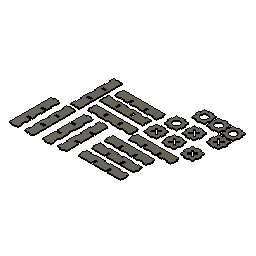
Verkefni2 (Autodesk Fusion 360 design; units mm, degrees)
Autodesk Fusion 360 part; units mm, degrees
note: some values were not read from the file. Chosen so that the rebuilt part matches the saved one: which bodies a step acts on. Set by a fixed rule: which sketch regions a step uses.
(part 1 of 6)
sketch "Rammi_lengd1_sketch" plane through (0, 0, 0) normal (1, 0, 0) x (0, 1, 0)
  line L0 (0, 0) -> (200, 0)
  line L1 (200, 0) -> (200, 40)
  line L2 (200, 40) -> (0, 40)
  line L3 (0, 40) -> (0, 0)
  dimension "d3" = 40
  dimension "d4" = 200
  constraint horizontal L0
  constraint vertical L1
  constraint horizontal L2
  constraint vertical L3
  constraint coincident L0.start L3.end
  measures "d3" distance of L0.start L2.end
  measures "d4" distance of L0.start L0.end
extrude "Extrude1" add sketch "Rammi_lengd1_sketch" along normal blind 4 makes body 1
sketch "V_Fingur_haed_sketch" plane through (0, 0, 0) normal (0, -1, 0) x (1, 0, 0)
  line L0 (0, 40) -> (0, 0)
  line L1 (0, 0) -> (4, 0)
  line L2 (4, 0) -> (4, 40)
  line L3 (4, 40) -> (0, 40)
  line L4 (0, 8) -> (4, 8)
  line L5 (4, 8) -> (4, 16)
  line L6 (4, 16) -> (0, 16)
  line L7 (0, 16) -> (0, 8)
  dimension "d13" = 8
  dimension "d14" = 8
  constraint horizontal L4
  constraint vertical L5
  constraint horizontal L6
  constraint vertical L7
  constraint coincident L2 L5.end
  constraint coincident L0 L4.start
  measures "d13" distance of L4.end L5.end
  measures "d14" distance of L1.end L4.end
extrude "Extrude2" cut sketch "V_Fingur_haed_sketch" against normal blind 4 contours L0 L2 L4 L5 L6 L7 bodies 1
pattern_linear "R-Pattern1" count 2 spacing 16 along (0, 0, 1) of "Extrude2"
sketch "Rammi_breidd_sketch" plane through (0, 0, 0) normal (0, 1, 0) x (1, 0, 0)
  line L0 (0, 0) -> (200, 0)
  line L1 (200, 0) -> (200, -40)
  line L2 (200, -40) -> (0, -40)
  line L3 (0, -40) -> (0, 0)
  dimension "d21" = 200
  dimension "d22" = 40
  constraint horizontal L0
  constraint vertical L1
  constraint horizontal L2
  constraint vertical L3
  constraint coincident L0.start L3.end
  measures "d21" distance of L1.end L2.end
  measures "d22" distance of L0.end L1.end
extrude "Extrude3" add sketch "Rammi_breidd_sketch" along normal blind 4 separate body makes body 2
combine "Combine1" operation cut target body 2 tool bodies 1 keep tools
extrude "Extrude4" add 1 faces at (4, 134.6667, 18.6667) along direction (-1, 0, 0) blind 4 from surface at -196 separate body on bodies 1 makes body 3
combine "Combine2" operation cut target body 2 tool bodies 3 keep tools
extrude "Extrude6" add 1 faces at (68, 4, 34.6667) along direction (0, -1, 0) blind 4 from surface at -196 separate body on bodies 2 makes body 4
combine "Combine4" operation cut target body 1 tool bodies 4 keep tools
combine "Combine7" operation cut target body 3 tool bodies 4 keep tools
sketch "got_a_hlidum1" plane through (0, 0, 0) normal (-1, 0, 0) x (0, -1, 0)
  line L0 (-196, 8) -> (-200, 8)
  line L1 (-200, 8) -> (-200, 0)
  line L2 (-200, 0) -> (0, 0)
  line L3 (0, 0) -> (0, 8)
  line L4 (0, 8) -> (-4, 8)
  line L5 (-4, 8) -> (-4, 16)
  line L6 (-4, 16) -> (0, 16)
  line L7 (0, 16) -> (0, 24)
  line L8 (0, 24) -> (-4, 24)
  line L9 (-4, 24) -> (-4, 32)
  line L10 (-4, 32) -> (0, 32)
  line L11 (0, 32) -> (0, 40)
  line L12 (0, 40) -> (-200, 40)
  line L13 (-200, 40) -> (-200, 32)
  line L14 (-200, 32) -> (-196, 32)
  line L15 (-196, 32) -> (-196, 24)
  line L16 (-196, 24) -> (-200, 24)
  line L17 (-200, 24) -> (-200, 16)
  line L18 (-200, 16) -> (-196, 16)
  line L19 (-196, 16) -> (-196, 8)
  line L20 (-137.3333, 28) -> (-129.3333, 28)
  line L21 (-129.3333, 28) -> (-129.3333, 12)
  line L22 (-129.3333, 12) -> (-137.3333, 12)
  line L23 (-137.3333, 12) -> (-137.3333, 28)
  dimension "d53" = 8
  dimension "d54" = 16
  dimension "d55" = 12
  dimension "d57" = 62.6667
  constraint horizontal L20
  constraint vertical L21
  constraint horizontal L22
  constraint vertical L23
  measures "d53" distance of L20.start L20.end
  measures "d54" distance of L20.end L21.end
  measures "d55" distance of L2 L22
  measures "d57" distance of L17 L23
extrude "Extrude8" cut sketch "got_a_hlidum1" against normal blind 4 contours L20 L21 L22 L23 bodies 1
sketch "got_a_hlidum2" plane through (0, 0, 0) normal (0, -1, 0) x (1, 0, 0)
  line L0 (196, 0) -> (196, 8)
  line L1 (196, 8) -> (200, 8)
  line L2 (200, 8) -> (200, 16)
  line L3 (200, 16) -> (196, 16)
  line L4 (196, 16) -> (196, 24)
  line L5 (196, 24) -> (200, 24)
  line L6 (200, 24) -> (200, 32)
  line L7 (200, 32) -> (196, 32)
  line L8 (196, 32) -> (196, 40)
  line L9 (196, 40) -> (4, 40)
  line L10 (4, 40) -> (4, 32)
  line L11 (4, 32) -> (0, 32)
  line L12 (0, 32) -> (0, 24)
  line L13 (0, 24) -> (4, 24)
  line L14 (4, 24) -> (4, 16)
  line L15 (4, 16) -> (0, 16)
  line L16 (0, 16) -> (0, 8)
  line L17 (0, 8) -> (4, 8)
  line L18 (4, 8) -> (4, 0)
  line L19 (4, 0) -> (196, 0)
  line L20 (62.6667, 28) -> (70.6667, 28)
  line L21 (70.6667, 28) -> (70.6667, 12)
  line L22 (70.6667, 12) -> (62.6667, 12)
  line L23 (62.6667, 12) -> (62.6667, 28)
  dimension "d68" = 8
  dimension "d69" = 16
  dimension "d70" = 62.6667
  dimension "d71" = 12
  constraint horizontal L20
  constraint vertical L21
  constraint horizontal L22
  constraint vertical L23
  measures "d68" distance of L20.start L20.end
  measures "d69" distance of L20.start L22.end
  measures "d70" distance of L16 L23
  measures "d71" distance of L9 L20
pattern_linear "R-Pattern3" count 2 spacing 66.6667 along (0, -1, 0) of "Extrude8"
extrude "Extrude9" cut sketch "got_a_hlidum2" against normal blind 4 contours L20 L21 L22 L23 bodies 2
pattern_linear "R-Pattern4" count 2 spacing 66.6667 along (1, 0, 0) of "Extrude9"
sketch "got_a_hlidum3" plane through (200, 0, 0) normal (1, 0, 0) x (0, 1, 0)
  line L0 (200, 8) -> (196, 8)
  line L1 (196, 8) -> (196, 16)
  line L2 (196, 16) -> (200, 16)
  line L3 (200, 16) -> (200, 24)
  line L4 (200, 24) -> (196, 24)
  line L5 (196, 24) -> (196, 32)
  line L6 (196, 32) -> (200, 32)
  line L7 (200, 40) -> (0, 40)
  line L8 (0, 40) -> (0, 32)
  line L9 (0, 32) -> (4, 32)
  line L10 (4, 32) -> (4, 24)
  line L11 (4, 24) -> (0, 24)
  line L12 (0, 24) -> (0, 16)
  line L13 (0, 16) -> (4, 16)
  line L14 (4, 16) -> (4, 8)
  line L15 (4, 8) -> (0, 8)
  line L16 (0, 8) -> (0, 0)
  line L17 (0, 0) -> (200, 0)
  line L18 (200, 0) -> (200, 8)
  line L19 (62.6667, 28) -> (70.6667, 28)
  line L20 (70.6667, 28) -> (70.6667, 12)
  line L21 (70.6667, 12) -> (62.6667, 12)
  line L22 (62.6667, 12) -> (62.6667, 28)
  line L23 (200, 32) -> (200, 40)
  dimension "d78" = 8
  dimension "d80" = 62.6667
  dimension "d178" = 16
  dimension "d179" = 12
  constraint horizontal L19
  constraint vertical L20
  constraint horizontal L21
  constraint vertical L22
  measures "d78" distance of L19.start L19.end
  measures "d80" distance of L12 L22
  measures "d178" distance of L19.start L21.end
  measures "d179" distance of L17 L21.end
extrude "Extrude10" cut sketch "got_a_hlidum3" against normal blind 4 contours L19 L20 L21 L22 bodies 3
pattern_linear "R-Pattern5" count 2 spacing 66.6667 along (0, 1, 0) of "Extrude10"
sketch "got_a_hlidum4" plane through (0, 200, 0) normal (0, 1, 0) x (-1, 0, 0)
  line L0 (-200, 8) -> (-196, 8)
  line L1 (-196, 8) -> (-196, 0)
  line L2 (-196, 0) -> (-4, 0)
  line L3 (-4, 0) -> (-4, 8)
  line L4 (-4, 8) -> (0, 8)
  line L5 (0, 8) -> (0, 16)
  line L6 (0, 16) -> (-4, 16)
  line L7 (-4, 16) -> (-4, 24)
  line L8 (-4, 24) -> (0, 24)
  line L9 (0, 24) -> (0, 32)
  line L10 (0, 32) -> (-4, 32)
  line L11 (-4, 32) -> (-4, 40)
  line L12 (-4, 40) -> (-196, 40)
  line L13 (-196, 40) -> (-196, 32)
  line L14 (-196, 32) -> (-200, 32)
  line L15 (-200, 32) -> (-200, 24)
  line L16 (-200, 24) -> (-196, 24)
  line L17 (-196, 24) -> (-196, 16)
  line L18 (-196, 16) -> (-200, 16)
  line L19 (-200, 16) -> (-200, 8)
  line L20 (-137.3333, 28) -> (-129.3333, 28)
  line L21 (-129.3333, 28) -> (-129.3333, 12)
  line L22 (-129.3333, 12) -> (-137.3333, 12)
  line L23 (-137.3333, 12) -> (-137.3333, 28)
  dimension "d92" = 8
  dimension "d93" = 12
  dimension "d94" = 16
  dimension "d95" = 62.6667
  constraint horizontal L20
  constraint vertical L21
  constraint horizontal L22
  constraint vertical L23
  measures "d92" distance of L20.start L20.end
  measures "d93" distance of L12 L20.start
  measures "d94" distance of L20.start L22.end
  measures "d95" distance of L19 L22.end
extrude "Extrude11" cut sketch "got_a_hlidum4" against normal blind 4 contours L20 L21 L22 L23 bodies 4
pattern_linear "R-Pattern6" count 2 spacing 66.6667 along (-1, 0, 0) of "Extrude11"
sketch "Millihlid_breidd_11_Sketch" plane through (0, 0, 0) normal (0, 1, 0) x (1, 0, 0)
  line L0 (62.6667, -40) -> (66.6667, -40)
  line L1 (66.6667, -40) -> (66.6667, 0)
  line L2 (66.6667, 0) -> (62.6667, 0)
  line L3 (62.6667, 0) -> (62.6667, -40)
  dimension "d103" = 4
  dimension "d104" = 62.6667
  dimension "d134" = 40
  dimension "d135" = 40
  constraint horizontal L0
  constraint vertical L1
  constraint horizontal L2
  constraint vertical L3
  measures "d103" distance of L0.start L0.end
  measures "d104" distance of origin L2.end
  measures "d134" distance of L0.end L1.end
  measures "d135" vertical distance of L0.end L2.end
extrude "Extrude12" add sketch "Millihlid_breidd_11_Sketch" along normal blind 200 separate body makes body 5
combine "Combine10" operation cut target body 5 tool bodies 2 keep tools
combine "Combine11" operation cut target body 5 tool bodies 4 keep tools
sketch "Millihlid_breidd_12_sketch" plane through (0, 0, 0) normal (0, -1, 0) x (1, 0, 0)
  line L0 (137.3333, 28) -> (137.3333, 12)
  line L1 (137.3333, 12) -> (129.3333, 12)
  line L2 (129.3333, 12) -> (129.3333, 28)
  line L3 (129.3333, 28) -> (137.3333, 28)
  line L4 (70.6667, 28) -> (70.6667, 12)
  line L5 (70.6667, 12) -> (62.6667, 12)
  line L6 (62.6667, 12) -> (62.6667, 28)
  line L7 (62.6667, 28) -> (70.6667, 28)
  line L8 (196, 0) -> (196, 8)
  line L9 (196, 8) -> (200, 8)
  line L10 (200, 8) -> (200, 16)
  line L11 (200, 16) -> (196, 16)
  line L12 (196, 16) -> (196, 24)
  line L13 (196, 24) -> (200, 24)
  line L14 (200, 24) -> (200, 32)
  line L15 (200, 32) -> (196, 32)
  line L16 (196, 32) -> (196, 40)
  line L17 (196, 40) -> (4, 40)
  line L18 (4, 40) -> (4, 32)
  line L19 (4, 32) -> (0, 32)
  line L20 (0, 32) -> (0, 24)
  line L21 (0, 24) -> (4, 24)
  line L22 (4, 24) -> (4, 16)
  line L23 (4, 16) -> (0, 16)
  line L24 (0, 16) -> (0, 8)
  line L25 (0, 8) -> (4, 8)
  line L26 (4, 8) -> (4, 0)
  line L27 (4, 0) -> (196, 0)
  line L28 (66.6667, 40) -> (70.6667, 40)
  line L29 (70.6667, 40) -> (70.6667, 0)
  line L30 (70.6667, 0) -> (66.6667, 0)
  line L31 (66.6667, 0) -> (66.6667, 40)
  dimension "d113" = 40
  dimension "d114" = 4
  dimension "d115" = 66.6667
  constraint horizontal L28
  constraint vertical L29
  constraint horizontal L30
  constraint vertical L31
  constraint coincident L17 L28.start
  measures "d113" distance of L28.end L29.end
  measures "d114" distance of L28.start L28.end
  measures "d115" distance of origin L30.end
extrude "Extrude13" add sketch "Millihlid_breidd_12_sketch" against normal blind 200 separate body contours L4 L5 L7 L29 L31 | L7 L17 L28 L29 L31 | L5 L27 L29 L30 L31 makes body 6
combine "Combine12" operation cut target body 6 tool bodies 2 keep tools
combine "Combine13" operation cut target body 6 tool bodies 4 keep tools
sketch "Millihlid_breidd_22_s" plane through (0, 0, 0) normal (0, 1, 0) x (1, 0, 0)
  line L0 (129.3333, -40) -> (133.3333, -40)
  line L1 (133.3333, -40) -> (133.3333, 0)
  line L2 (133.3333, 0) -> (129.3333, 0)
  line L3 (129.3333, 0) -> (129.3333, -40)
  dimension "d124" = 4
  dimension "d125" = 40
  dimension "d126" = 129.3333
  constraint horizontal L0
  constraint vertical L1
  constraint horizontal L2
  constraint vertical L3
  measures "d124" distance of L1.end L2.end
  measures "d125" distance of L0.start L2.end
  measures "d126" distance of origin L2.end
extrude "Extrude14" add sketch "Millihlid_breidd_22_s" along normal blind 200 separate body makes body 7
combine "Combine14" operation cut target body 7 tool bodies 2 keep tools
combine "Combine15" operation cut target body 7 tool bodies 4 keep tools
sketch "Millihlid_breidd_21_sketch" plane through (0, 0, 0) normal (0, 1, 0) x (1, 0, 0)
  line L0 (133.3333, -40) -> (137.3333, -40)
  line L1 (137.3333, -40) -> (137.3333, 0)
  line L2 (137.3333, 0) -> (133.3333, 0)
  line L3 (133.3333, 0) -> (133.3333, -40)
  point P0 (200, 0)
  dimension "d129" = 40
  dimension "d130" = 4
  dimension "d131" = 62.6667
  constraint horizontal L0
  constraint vertical L1
  constraint horizontal L2
  constraint vertical L3
  measures "d129" distance of L0.end L1.end
  measures "d130" distance of L1.end L2.end
  measures "d131" distance of L1.end P0
extrude "Extrude15" add sketch "Millihlid_breidd_21_sketch" along normal blind 200 separate body makes body 8
combine "Combine16" operation cut target body 8 tool bodies 2 keep tools
combine "Combine17" operation cut target body 8 tool bodies 4 keep tools
sketch "Sketch38" plane through (62.6667, 0, 0) normal (-1, 0, 0) x (0, -1, 0)
  line L0 (-196, 0) -> (-4, 0)
  line L1 (-4, 0) -> (-4, 12)
  line L2 (-4, 12) -> (0, 12)
  line L3 (0, 12) -> (0, 28)
  line L4 (-4, 40) -> (-196, 40)
  line L5 (-137.3333, 0) -> (-129.3333, 0)
  line L6 (-129.3333, 0) -> (-129.3333, 20)
  line L7 (-129.3333, 20) -> (-137.3333, 20)
  line L8 (-137.3333, 20) -> (-137.3333, 0)
  line L9 (0, 28) -> (-4, 28)
  line L10 (-4, 28) -> (-4, 40)
  line L11 (-196, 12) -> (-196, 0)
  line L12 (-196, 28) -> (-200, 28)
  line L13 (-200, 28) -> (-200, 12)
  line L14 (-200, 12) -> (-196, 12)
  line L15 (-196, 40) -> (-196, 28)
  dimension "d148" = 20
  dimension "d149" = 8
  dimension "d199" = 58.6667
  constraint horizontal L5
  constraint vertical L6
  constraint horizontal L7
  constraint vertical L8
  constraint coincident L0 L5.start
  measures "d148" distance of L5.start L7.end
  measures "d149" distance of L6.end L7.end
  measures "d199" distance of L5.start L0.start
extrude "Extrude18" cut sketch "Sketch38" against normal blind 8 contours L0 L5 L6 L7 L8 bodies 5 6
pattern_linear "R-Pattern7" count 2 spacing 66.6667 along (0, -1, 0) of "Extrude18"
sketch "Festigot_millihlid2" plane through (137.3333, 0, 0) normal (1, 0, 0) x (0, 1, 0)
  line L0 (196, 0) -> (196, 12)
  line L1 (196, 12) -> (200, 12)
  line L2 (200, 12) -> (200, 28)
  line L3 (196, 40) -> (4, 40)
  line L4 (0, 28) -> (0, 12)
  line L5 (0, 12) -> (4, 12)
  line L6 (4, 40) -> (4, 28)
  line L7 (4, 0) -> (196, 0)
  line L8 (62.6667, 0) -> (70.6667, 0)
  line L9 (70.6667, 0) -> (70.6667, 20)
  line L10 (70.6667, 20) -> (62.6667, 20)
  line L11 (62.6667, 20) -> (62.6667, 0)
  line L12 (200, 28) -> (196, 28)
  line L13 (4, 28) -> (0, 28)
  line L14 (196, 28) -> (196, 40)
  line L15 (4, 12) -> (4, 0)
  dimension "d157" = 8
  dimension "d158" = 20
  dimension "d159" = 62.6667
  constraint horizontal L8
  constraint vertical L9
  constraint horizontal L10
  constraint vertical L11
  constraint coincident L7 L8.start
  measures "d157" distance of L9.end L10.end
  measures "d158" distance of L8.start L10.end
  measures "d159" distance of origin L8.start
extrude "Extrude19" cut sketch "Festigot_millihlid2" against normal blind 8 contours L7 L8 L9 L10 L11 bodies 8
pattern_linear "R-Pattern8" count 2 spacing 66.6667 along (0, 1, 0) of "Extrude19"
sketch "Sketch49" plane through (129.3333, 0, 0) normal (-1, 0, 0) x (0, -1, 0)
  line L0 (-196, 12) -> (-196, 0)
  line L1 (-196, 0) -> (-4, 0)
  line L2 (-4, 0) -> (-4, 12)
  line L3 (-4, 12) -> (0, 12)
  line L4 (0, 12) -> (0, 28)
  line L5 (0, 28) -> (-4, 28)
  line L6 (-4, 28) -> (-4, 40)
  line L7 (-4, 40) -> (-196, 40)
  line L8 (-196, 40) -> (-196, 28)
  line L9 (-196, 28) -> (-200, 28)
  line L10 (-200, 28) -> (-200, 12)
  line L11 (-200, 12) -> (-196, 12)
  line L12 (-70.6667, 0) -> (-62.6667, 0)
  line L13 (-62.6667, 0) -> (-62.6667, 20)
  line L14 (-62.6667, 20) -> (-70.6667, 20)
  line L15 (-70.6667, 20) -> (-70.6667, 0)
  dimension "d200" = 20
  dimension "d201" = 8
  dimension "d202" = 58.6667
  constraint horizontal L12
  constraint vertical L13
  constraint horizontal L14
  constraint vertical L15
  constraint coincident L1 L12.start
  measures "d200" distance of L12.end L13.end
  measures "d201" distance of L13.end L14.end
  measures "d202" distance of L1.end L12.end
extrude "Extrude24" cut sketch "Sketch49" against normal blind 4 contours L1 L12 L13 L14 L15 bodies 7
pattern_linear "R-Pattern9" count 2 spacing 66.6667 along (0, 1, 0) of "Extrude24"
sketch "millihlid_lengd" plane through (200, 0, 0) normal (1, 0, 0) x (0, 1, 0)
  line L0 (137.3333, 28) -> (137.3333, 12)
  line L1 (137.3333, 12) -> (129.3333, 12)
  line L2 (129.3333, 12) -> (129.3333, 28)
  line L3 (70.6667, 28) -> (70.6667, 12)
  line L4 (70.6667, 12) -> (62.6667, 12)
  line L5 (62.6667, 12) -> (62.6667, 28)
  line L6 (200, 8) -> (196, 8)
  line L7 (196, 8) -> (196, 16)
  line L8 (196, 16) -> (200, 16)
  line L9 (200, 16) -> (200, 24)
  line L10 (200, 24) -> (196, 24)
  line L11 (196, 24) -> (196, 32)
  line L12 (196, 32) -> (200, 32)
  line L13 (200, 40) -> (0, 40)
  line L14 (0, 40) -> (0, 32)
  line L15 (0, 32) -> (4, 32)
  line L16 (4, 32) -> (4, 24)
  line L17 (4, 24) -> (0, 24)
  line L18 (0, 24) -> (0, 16)
  line L19 (0, 16) -> (4, 16)
  line L20 (4, 16) -> (4, 8)
  line L21 (4, 8) -> (0, 8)
  line L22 (0, 8) -> (0, 0)
  line L23 (0, 0) -> (200, 0)
  line L24 (200, 0) -> (200, 8)
  line L25 (62.6667, 40) -> (66.6667, 40)
  line L26 (66.6667, 40) -> (66.6667, 0)
  line L27 (66.6667, 0) -> (62.6667, 0)
  line L28 (62.6667, 0) -> (62.6667, 40)
  line L29 (200, 32) -> (200, 40)
  line L30 (129.3333, 28) -> (137.3333, 28)
  line L31 (62.6667, 28) -> (70.6667, 28)
  dimension "d166" = 4
  dimension "d167" = 40
  dimension "d168" = 62.6667
  constraint horizontal L25
  constraint vertical L26
  constraint horizontal L27
  constraint vertical L28
  constraint coincident L13 L25.start
  measures "d166" distance of L25.start L25.end
  measures "d167" distance of L25.start L27.end
  measures "d168" distance of L22.end L27.end
extrude "Extrude20" add sketch "millihlid_lengd" against normal blind 200 separate body contours L13 L25 L26 L28 L31 | L4 L5 L26 L28 L31 | L4 L23 L26 L27 L28 makes body 9
combine "Combine28" operation cut target body 9 tool bodies 8 keep tools
combine "Combine27" operation cut target body 9 tool bodies 3 keep tools
combine "Combine29" operation cut target body 9 tool bodies 7 keep tools
combine "Combine30" operation cut target body 9 tool bodies 6 keep tools
combine "Combine31" operation cut target body 9 tool bodies 5 keep tools
sketch "millihlid_lengd12" plane through (200, 0, 0) normal (1, 0, 0) x (0, 1, 0)
  line L0 (137.3333, 28) -> (137.3333, 12)
  line L1 (137.3333, 12) -> (129.3333, 12)
  line L2 (129.3333, 12) -> (129.3333, 28)
  line L3 (70.6667, 28) -> (70.6667, 12)
  line L4 (70.6667, 12) -> (62.6667, 12)
  line L5 (62.6667, 12) -> (62.6667, 28)
  line L6 (200, 8) -> (196, 8)
  line L7 (196, 8) -> (196, 16)
  line L8 (196, 16) -> (200, 16)
  line L9 (200, 16) -> (200, 24)
  line L10 (200, 24) -> (196, 24)
  line L11 (196, 24) -> (196, 32)
  line L12 (196, 32) -> (200, 32)
  line L13 (200, 40) -> (0, 40)
  line L14 (0, 40) -> (0, 32)
  line L15 (0, 32) -> (4, 32)
  line L16 (4, 32) -> (4, 24)
  line L17 (4, 24) -> (0, 24)
  line L18 (0, 24) -> (0, 16)
  line L19 (0, 16) -> (4, 16)
  line L20 (4, 16) -> (4, 8)
  line L21 (4, 8) -> (0, 8)
  line L22 (0, 8) -> (0, 0)
  line L23 (0, 0) -> (200, 0)
  line L24 (200, 0) -> (200, 8)
  line L25 (66.6667, 40) -> (70.6667, 40)
  line L26 (70.6667, 40) -> (70.6667, 0)
  line L27 (70.6667, 0) -> (66.6667, 0)
  line L28 (66.6667, 0) -> (66.6667, 40)
  line L29 (200, 32) -> (200, 40)
  line L30 (129.3333, 28) -> (137.3333, 28)
  line L31 (62.6667, 28) -> (70.6667, 28)
  dimension "d171" = 4
  dimension "d172" = 40
  dimension "d173" = 66.6667
  constraint horizontal L25
  constraint vertical L26
  constraint horizontal L27
  constraint vertical L28
  constraint coincident L13 L25.start
  measures "d171" distance of L25.start L25.end
  measures "d172" distance of L25.end L26.end
  measures "d173" distance of L22.end L27.end
combine "Combine32" operation cut target body 9 tool bodies 1 keep tools
extrude "Extrude21" add sketch "millihlid_lengd12" against normal blind 200 separate body contours L13 L25 L26 L28 L31 | L3 L4 L26 L28 L31 | L4 L23 L26 L27 L28 makes body 10
combine "Combine47" operation cut target body 10 tool bodies 3 7 6 5 1 keep tools
combine "Combine33" operation cut target body 10 tool bodies 1 keep tools
combine "Combine34" operation cut target body 10 tool bodies 5 keep tools
combine "Combine35" operation cut target body 10 tool bodies 6 keep tools
combine "Combine36" operation cut target body 10 tool bodies 7 keep tools
combine "Combine37" operation cut target body 10 tool bodies 8 keep tools
combine "Combine38" operation cut target body 10 tool bodies 3 keep tools
sketch "Millihlid_lengd21" plane through (0, 0, 0) normal (1, 0, 0) x (0, 1, 0)
  line L0 (137.3333, 0) -> (133.3333, 0)
  line L1 (133.3333, 0) -> (133.3333, 40)
  line L2 (133.3333, 40) -> (137.3333, 40)
  line L3 (137.3333, 40) -> (137.3333, 0)
  point P0 (200, 0)
  dimension "d180" = 40
  dimension "d181" = 4
  dimension "d182" = 62.6667
  constraint horizontal L0
  constraint vertical L1
  constraint horizontal L2
  constraint vertical L3
  measures "d180" distance of L0.start L2.end
  measures "d181" distance of L0.start L0.end
  measures "d182" distance of L0.start P0
extrude "Extrude22" add sketch "Millihlid_lengd21" along normal blind 200 separate body makes body 11
combine "Combine44" operation cut target body 11 tool bodies 1 6 5 8 7 3 keep tools
sketch "Sketch43" plane through (0, 0, 0) normal (1, 0, 0) x (0, 1, 0)
  line L0 (133.3333, 40) -> (129.3333, 40)
  line L1 (129.3333, 40) -> (129.3333, 0)
  line L2 (129.3333, 0) -> (133.3333, 0)
  line L3 (133.3333, 0) -> (133.3333, 40)
  point P0 (200, 0)
  dimension "d185" = 40
  dimension "d186" = 4
  dimension "d187" = 66.6667
  constraint horizontal L0
  constraint vertical L1
  constraint horizontal L2
  constraint vertical L3
  measures "d185" distance of L0.start L2.end
  measures "d186" distance of L0.start L0.end
  measures "d187" distance of L2.end P0
combine "Combine43" operation cut target body 11 tool bodies 8 keep tools
extrude "Extrude23" add sketch "Sketch43" along normal blind 200 separate body makes body 12
combine "Combine45" operation cut target body 12 tool bodies 1 5 6 7 8 3 keep tools
sketch "toppur_lengd sketch" plane through (0, 0, 40) normal (0, 0, 1) x (-1, 0, 0)
  line L0 (-200, 0) -> (-200, -200)
  line L1 (-200, -200) -> (-196, -200)
  line L2 (-196, -200) -> (-196, 0)
  line L3 (-196, 0) -> (-200, 0)
  line L4 (-196, -44.4444) -> (-200, -44.4444)
  line L5 (-200, -44.4444) -> (-200, -22.2222)
  line L6 (-200, -22.2222) -> (-196, -22.2222)
  line L7 (-196, -22.2222) -> (-196, -44.4444)
  dimension "d194" = 4
  dimension "d196" = 22.2222
  dimension "d197" = 22.2222
  constraint horizontal L4
  constraint vertical L5
  constraint horizontal L6
  constraint vertical L7
  constraint coincident L2 L4.start
  measures "d194" distance of L4.start L4.end
  measures "d196" distance of L4.end L5.end
  measures "d197" distance of L0.start L5.end
extrude "Extrude25" cut sketch "toppur_lengd sketch" against normal blind 4 contours L0 L2 L4 L5 L6 L7 bodies 3
pattern_linear "R-Pattern10" count 3 spacing 66.6667 along (0, 1, 0) of "Extrude25"
sketch "toppur_breidd_sketch" plane through (0, 0, 40) normal (0, 0, 1) x (-1, 0, 0)
  line L0 (-196, -200) -> (-4, -200)
  line L1 (-4, -200) -> (-4, -196)
  line L2 (-4, -196) -> (-196, -196)
  line L3 (-196, -196) -> (-196, -200)
  line L4 (-177.7778, -196) -> (-155.5556, -196)
  line L5 (-155.5556, -196) -> (-155.5556, -200)
  line L6 (-155.5556, -200) -> (-177.7778, -200)
  line L7 (-177.7778, -200) -> (-177.7778, -196)
  point P0 (-200, -200)
  dimension "d215" = 4
  dimension "d216" = 22.2222
  dimension "d217" = 22.2222
  constraint horizontal L4
  constraint vertical L5
  constraint horizontal L6
  constraint vertical L7
  constraint coincident L2 L4.start
  measures "d215" distance of L4.end L5.end
  measures "d216" distance of L5.end L6.end
  measures "d217" distance of L6.end P0
extrude "Extrude26" cut sketch "toppur_breidd_sketch" against normal blind 4 contours L0 L2 L4 L5 L6 L7 bodies 4
pattern_linear "R-Pattern11" count 3 spacing 66.6667 along (-1, 0, 0) of "Extrude26"
sketch "toppur_lengd_sketch_2" plane through (0, 0, 40) normal (0, 0, 1) x (-1, 0, 0)
  line L0 (0, -200) -> (0, 0)
  line L1 (0, 0) -> (-4, 0)
  line L2 (-4, 0) -> (-4, -200)
  line L3 (-4, -200) -> (0, -200)
  line L4 (-4, -177.7778) -> (0, -177.7778)
  line L5 (0, -177.7778) -> (0, -155.5556)
  line L6 (0, -155.5556) -> (-4, -155.5556)
  line L7 (-4, -155.5556) -> (-4, -177.7778)
  dimension "d225" = 4
  dimension "d226" = 22.2222
  dimension "d227" = 22.2222
  constraint horizontal L4
  constraint vertical L5
  constraint horizontal L6
  constraint vertical L7
  constraint coincident L2 L4.start
  measures "d225" distance of L5.end L6.end
  measures "d226" distance of L4.end L5.end
  measures "d227" distance of L0.start L4.end
extrude "Extrude27" cut sketch "toppur_lengd_sketch_2" against normal blind 4 contours L0 L2 L4 L5 L6 L7 bodies 1
pattern_linear "R-Pattern12" count 3 spacing 66.6667 along (0, -1, 0) of "Extrude27"
sketch "Sketch52" plane through (0, 0, 40) normal (0, 0, 1) x (-1, 0, 0)
  line L0 (-62.6667, -129.3333) -> (-62.6667, -133.3333)
  line L1 (-62.6667, -133.3333) -> (-4, -133.3333)
  line L2 (-4, -133.3333) -> (-4, -129.3333)
  line L3 (-4, -129.3333) -> (-62.6667, -129.3333)
  line L4 (-22.2222, -4) -> (-44.4444, -4)
  line L5 (-44.4444, -4) -> (-44.4444, 0)
  line L6 (-44.4444, 0) -> (-22.2222, 0)
  line L7 (-22.2222, 0) -> (-22.2222, -4)
  dimension "d234" = 4
  dimension "d235" = 22.2222
  dimension "d236" = 22.2222
  constraint horizontal L4
  constraint vertical L5
  constraint horizontal L6
  constraint vertical L7
  measures "d234" distance of L4.start L6.end
  measures "d235" distance of L5.end L6.end
  measures "d236" distance of origin L6.end
extrude "Extrude28" cut sketch "Sketch52" against normal blind 4 contours L4 L5 L6 L7 bodies 2
pattern_linear "R-Pattern13" count 3 spacing 66.6667 along (1, 0, 0) of "Extrude28"
sketch "Sketch54" plane through (0, 0, 40) normal (0, 0, 1) x (-1, 0, 0)
  line L0 (-62.6667, -133.3333) -> (-62.6667, -137.3333)
  line L1 (-62.6667, -137.3333) -> (-4, -137.3333)
  line L2 (-4, -137.3333) -> (-4, -133.3333)
  line L3 (-4, -133.3333) -> (-62.6667, -133.3333)
  line L4 (-22.2222, -137.3333) -> (-44.4444, -137.3333)
  line L5 (-44.4444, -137.3333) -> (-44.4444, -129.3333)
  line L6 (-44.4444, -129.3333) -> (-22.2222, -129.3333)
  line L7 (-22.2222, -129.3333) -> (-22.2222, -137.3333)
  line L8 (0, -155.5556) -> (0, -111.1111)
  dimension "d245" = 8
  dimension "d246" = 22.2222
  dimension "d247" = 22.2222
  constraint horizontal L4
  constraint vertical L5
  constraint horizontal L6
  constraint vertical L7
  constraint coincident L1 L4.start
  measures "d245" distance of L4.start L6.end
  measures "d246" distance of L5.end L6.end
  measures "d247" distance of L6.end L8
extrude "Extrude29" cut sketch "Sketch54" against normal blind 4 contours L3 L5 L6 L7 | L1 L3 L4 L5 L7 bodies 11 12
pattern_linear "R-Pattern14" count 3 spacing 66.6667 along (1, 0, 0) of "Extrude29"
sketch "Sketch55" plane through (0, 0, 40) normal (0, 0, 1) x (-1, 0, 0)
  line L0 (-196, -62.6667) -> (-196, -66.6667)
  line L1 (-196, -66.6667) -> (-137.3333, -66.6667)
  line L2 (-137.3333, -66.6667) -> (-137.3333, -62.6667)
  line L3 (-137.3333, -62.6667) -> (-196, -62.6667)
  line L4 (-155.5556, -62.6667) -> (-177.7778, -62.6667)
  line L5 (-177.7778, -62.6667) -> (-177.7778, -70.6667)
  line L6 (-177.7778, -70.6667) -> (-155.5556, -70.6667)
  line L7 (-155.5556, -70.6667) -> (-155.5556, -62.6667)
  line L8 (-200, -44.4444) -> (-200, -88.8889)
  dimension "d254" = 8
  dimension "d255" = 22.2222
  dimension "d256" = 22.2222
  constraint horizontal L4
  constraint vertical L5
  constraint horizontal L6
  constraint vertical L7
  constraint coincident L3 L4.start
  measures "d254" distance of L4.end L5.end
  measures "d255" distance of L5.end L6.end
  measures "d256" distance of L5.end L8
extrude "Extrude30" cut sketch "Sketch55" against normal blind 4 contours L1 L3 L4 L5 L7 | L1 L5 L6 L7 bodies 9 10
pattern_linear "R-Pattern15" count 3 spacing 66.6667 along (-1, 0, 0) of "Extrude30"
sketch "Sketch56" plane through (0, 0, 40) normal (0, 0, 1) x (-1, 0, 0)
  line L0 (-66.6667, -196) -> (-62.6667, -196)
  line L1 (-62.6667, -196) -> (-62.6667, -4)
  line L2 (-62.6667, -4) -> (-66.6667, -4)
  line L3 (-66.6667, -4) -> (-66.6667, -196)
  line L4 (-62.6667, -22.2222) -> (-70.6667, -22.2222)
  line L5 (-70.6667, -22.2222) -> (-70.6667, -44.4444)
  line L6 (-70.6667, -44.4444) -> (-62.6667, -44.4444)
  line L7 (-62.6667, -44.4444) -> (-62.6667, -22.2222)
  line L8 (-88.8889, 0) -> (-44.4444, 0)
  dimension "d263" = 8
  dimension "d264" = 22.2222
  dimension "d265" = 22.2222
  constraint horizontal L4
  constraint vertical L5
  constraint horizontal L6
  constraint vertical L7
  constraint coincident L1 L4.start
  measures "d263" distance of L4.start L4.end
  measures "d264" distance of L4.end L5.end
  measures "d265" distance of L4.start L8
extrude "Extrude31" cut sketch "Sketch56" against normal blind 4 contours L3 L4 L5 L6 | L1 L3 L4 L6 L7 bodies 5 6
pattern_linear "R-Pattern16" count 3 spacing 66.6667 along (0, 1, 0) of "Extrude31"
sketch "Sketch57" plane through (0, 0, 40) normal (0, 0, 1) x (-1, 0, 0)
  line L0 (-137.3333, -196) -> (-133.3333, -196)
  line L1 (-133.3333, -196) -> (-133.3333, -4)
  line L2 (-133.3333, -4) -> (-137.3333, -4)
  line L3 (-137.3333, -4) -> (-137.3333, -196)
  line L4 (-137.3333, -22.2222) -> (-129.3333, -22.2222)
  line L5 (-129.3333, -22.2222) -> (-129.3333, -44.4444)
  line L6 (-129.3333, -44.4444) -> (-137.3333, -44.4444)
  line L7 (-137.3333, -44.4444) -> (-137.3333, -22.2222)
  line L8 (-155.5556, 0) -> (-111.1111, 0)
  dimension "d272" = 8
  dimension "d273" = 22.2222
  dimension "d274" = 22.2222
  constraint horizontal L4
  constraint vertical L5
  constraint horizontal L6
  constraint vertical L7
  constraint coincident L3 L4.start
  measures "d272" distance of L5.end L6.end
  measures "d273" distance of L4.start L6.end
  measures "d274" distance of L4.start L8
extrude "Extrude32" cut sketch "Sketch57" against normal blind 4 contours L1 L3 L4 L6 L7 | L1 L4 L5 L6 bodies 7 8
pattern_linear "R-Pattern17" count 3 spacing 66.6667 along (0, 1, 0) of "Extrude32"
sketch "Sketch64" plane through (0, 0, 40) normal (0, 0, 1) x (-1, 0, 0)
  line L0 (-200, -88.8889) -> (-196, -88.8889)
  line L1 (-196, -88.8889) -> (-196, -44.4444)
  line L2 (-196, -44.4444) -> (-200, -44.4444)
  line L3 (-200, -44.4444) -> (-200, -88.8889)
  line L4 (0, -200) -> (-200, -200)
  line L5 (-200, -200) -> (-200, 0)
  line L6 (-200, 0) -> (0, 0)
  line L7 (0, 0) -> (0, -200)
  dimension "d295" = 200
  dimension "d296" = 200
  constraint horizontal L4
  constraint vertical L5
  constraint horizontal L6
  constraint vertical L7
  measures "d295" distance of L5.end L6.end
  measures "d296" distance of L4.end L5.end
extrude "Extrude34" add sketch "Sketch64" against normal blind 4 separate body contours L0 L1 L2 L4 L5 L6 L7 makes body 13
combine "Combine48" operation cut target body 13 tool bodies 12 11 10 9 8 7 6 5 4 3 2 1 keep tools
sketch "Sketch65" plane through (0, 0, 36) normal (0, 0, -1) x (1, 0, 0)
  line L0 (4, -177.7778) -> (4, -196)
  line L1 (4, -196) -> (22.2222, -196)
  line L2 (22.2222, -196) -> (22.2222, -200)
  line L3 (22.2222, -200) -> (44.4444, -200)
  line L4 (44.4444, -200) -> (44.4444, -196)
  line L5 (44.4444, -196) -> (62.6667, -196)
  line L6 (62.6667, -196) -> (62.6667, -177.7778)
  line L7 (62.6667, -177.7778) -> (70.6667, -177.7778)
  line L8 (70.6667, -177.7778) -> (70.6667, -196)
  line L9 (70.6667, -196) -> (88.8889, -196)
  line L10 (88.8889, -196) -> (88.8889, -200)
  line L11 (88.8889, -200) -> (111.1111, -200)
  line L12 (111.1111, -200) -> (111.1111, -196)
  line L13 (111.1111, -196) -> (129.3333, -196)
  line L14 (129.3333, -196) -> (129.3333, -177.7778)
  line L15 (129.3333, -177.7778) -> (137.3333, -177.7778)
  line L16 (137.3333, -177.7778) -> (137.3333, -196)
  line L17 (137.3333, -196) -> (155.5556, -196)
  line L18 (155.5556, -196) -> (155.5556, -200)
  line L19 (155.5556, -200) -> (177.7778, -200)
  line L20 (177.7778, -200) -> (177.7778, -196)
  line L21 (177.7778, -196) -> (196, -196)
  line L22 (196, -196) -> (196, -177.7778)
  line L23 (196, -177.7778) -> (200, -177.7778)
  line L24 (200, -177.7778) -> (200, -155.5556)
  line L25 (200, -155.5556) -> (196, -155.5556)
  line L26 (196, -155.5556) -> (196, -137.3333)
  line L27 (196, -137.3333) -> (177.7778, -137.3333)
  line L28 (177.7778, -137.3333) -> (177.7778, -129.3333)
  line L29 (177.7778, -129.3333) -> (196, -129.3333)
  line L30 (196, -129.3333) -> (196, -111.1111)
  line L31 (196, -111.1111) -> (200, -111.1111)
  line L32 (200, -111.1111) -> (200, -88.8889)
  line L33 (200, -88.8889) -> (196, -88.8889)
  line L34 (196, -88.8889) -> (196, -70.6667)
  line L35 (196, -70.6667) -> (177.7778, -70.6667)
  line L36 (177.7778, -70.6667) -> (177.7778, -62.6667)
  line L37 (177.7778, -62.6667) -> (196, -62.6667)
  line L38 (196, -62.6667) -> (196, -44.4444)
  line L39 (196, -44.4444) -> (200, -44.4444)
  line L40 (200, -44.4444) -> (200, -22.2222)
  line L41 (200, -22.2222) -> (196, -22.2222)
  line L42 (196, -22.2222) -> (196, -4)
  line L43 (196, -4) -> (177.7778, -4)
  line L44 (177.7778, -4) -> (177.7778, 0)
  line L45 (177.7778, 0) -> (155.5556, 0)
  line L46 (155.5556, 0) -> (155.5556, -4)
  line L47 (155.5556, -4) -> (137.3333, -4)
  line L48 (137.3333, -4) -> (137.3333, -22.2222)
  line L49 (137.3333, -22.2222) -> (129.3333, -22.2222)
  line L50 (129.3333, -22.2222) -> (129.3333, -4)
  line L51 (129.3333, -4) -> (111.1111, -4)
  line L52 (111.1111, -4) -> (111.1111, 0)
  line L53 (111.1111, 0) -> (88.8889, 0)
  line L54 (88.8889, 0) -> (88.8889, -4)
  line L55 (88.8889, -4) -> (70.6667, -4)
  line L56 (70.6667, -4) -> (70.6667, -22.2222)
  line L57 (70.6667, -22.2222) -> (62.6667, -22.2222)
  line L58 (62.6667, -22.2222) -> (62.6667, -4)
  line L59 (62.6667, -4) -> (44.4444, -4)
  line L60 (44.4444, -4) -> (44.4444, 0)
  line L61 (44.4444, 0) -> (22.2222, 0)
  line L62 (22.2222, 0) -> (22.2222, -4)
  line L63 (22.2222, -4) -> (4, -4)
  line L64 (4, -4) -> (4, -22.2222)
  line L65 (4, -22.2222) -> (0, -22.2222)
  line L66 (0, -22.2222) -> (0, -44.4444)
  line L67 (0, -44.4444) -> (4, -44.4444)
  line L68 (4, -44.4444) -> (4, -62.6667)
  line L69 (4, -62.6667) -> (22.2222, -62.6667)
  line L70 (22.2222, -62.6667) -> (22.2222, -70.6667)
  line L71 (22.2222, -70.6667) -> (4, -70.6667)
  line L72 (4, -70.6667) -> (4, -88.8889)
  line L73 (4, -88.8889) -> (0, -88.8889)
  line L74 (0, -88.8889) -> (0, -111.1111)
  line L75 (0, -111.1111) -> (4, -111.1111)
  line L76 (4, -111.1111) -> (4, -129.3333)
  line L77 (4, -129.3333) -> (22.2222, -129.3333)
  line L78 (22.2222, -129.3333) -> (22.2222, -137.3333)
  line L79 (22.2222, -137.3333) -> (4, -137.3333)
  line L80 (4, -137.3333) -> (4, -155.5556)
  line L81 (4, -155.5556) -> (0, -155.5556)
  line L82 (0, -155.5556) -> (0, -177.7778)
  line L83 (0, -177.7778) -> (4, -177.7778)
  line L84 (62.6667, -155.5556) -> (62.6667, -137.3333)
  line L85 (62.6667, -137.3333) -> (44.4444, -137.3333)
  line L86 (44.4444, -137.3333) -> (44.4444, -129.3333)
  line L87 (44.4444, -129.3333) -> (62.6667, -129.3333)
  line L88 (62.6667, -129.3333) -> (62.6667, -111.1111)
  line L89 (62.6667, -111.1111) -> (70.6667, -111.1111)
  line L90 (70.6667, -111.1111) -> (70.6667, -129.3333)
  line L91 (70.6667, -129.3333) -> (88.8889, -129.3333)
  line L92 (88.8889, -129.3333) -> (88.8889, -137.3333)
  line L93 (88.8889, -137.3333) -> (70.6667, -137.3333)
  line L94 (70.6667, -137.3333) -> (70.6667, -155.5556)
  line L95 (70.6667, -155.5556) -> (62.6667, -155.5556)
  line L96 (62.6667, -88.8889) -> (62.6667, -70.6667)
  line L97 (62.6667, -70.6667) -> (44.4444, -70.6667)
  line L98 (44.4444, -70.6667) -> (44.4444, -62.6667)
  line L99 (44.4444, -62.6667) -> (62.6667, -62.6667)
  line L100 (62.6667, -62.6667) -> (62.6667, -44.4444)
  line L101 (62.6667, -44.4444) -> (70.6667, -44.4444)
  line L102 (70.6667, -44.4444) -> (70.6667, -62.6667)
  line L103 (70.6667, -62.6667) -> (88.8889, -62.6667)
  line L104 (88.8889, -62.6667) -> (88.8889, -70.6667)
  line L105 (88.8889, -70.6667) -> (70.6667, -70.6667)
  line L106 (70.6667, -70.6667) -> (70.6667, -88.8889)
  line L107 (70.6667, -88.8889) -> (62.6667, -88.8889)
  line L108 (129.3333, -88.8889) -> (129.3333, -70.6667)
  line L109 (129.3333, -70.6667) -> (111.1111, -70.6667)
  line L110 (111.1111, -70.6667) -> (111.1111, -62.6667)
  line L111 (111.1111, -62.6667) -> (129.3333, -62.6667)
  line L112 (129.3333, -62.6667) -> (129.3333, -44.4444)
  line L113 (129.3333, -44.4444) -> (137.3333, -44.4444)
  line L114 (137.3333, -44.4444) -> (137.3333, -62.6667)
  line L115 (137.3333, -62.6667) -> (155.5556, -62.6667)
  line L116 (155.5556, -62.6667) -> (155.5556, -70.6667)
  line L117 (155.5556, -70.6667) -> (137.3333, -70.6667)
  line L118 (137.3333, -70.6667) -> (137.3333, -88.8889)
  line L119 (137.3333, -88.8889) -> (129.3333, -88.8889)
  line L120 (129.3333, -155.5556) -> (129.3333, -137.3333)
  line L121 (129.3333, -137.3333) -> (111.1111, -137.3333)
  line L122 (111.1111, -137.3333) -> (111.1111, -129.3333)
  line L123 (111.1111, -129.3333) -> (129.3333, -129.3333)
  line L124 (129.3333, -129.3333) -> (129.3333, -111.1111)
  line L125 (129.3333, -111.1111) -> (137.3333, -111.1111)
  line L126 (137.3333, -111.1111) -> (137.3333, -129.3333)
  line L127 (137.3333, -129.3333) -> (155.5556, -129.3333)
  line L128 (155.5556, -129.3333) -> (155.5556, -137.3333)
  line L129 (155.5556, -137.3333) -> (137.3333, -137.3333)
  line L130 (137.3333, -137.3333) -> (137.3333, -155.5556)
  line L131 (137.3333, -155.5556) -> (129.3333, -155.5556)
  line L132 (66.1667, -22.2222) -> (67.1667, -22.2222)
  line L133 (67.1667, -22.2222) -> (67.1667, -44.4444)
  line L134 (67.1667, -44.4444) -> (66.1667, -44.4444)
  line L135 (66.1667, -44.4444) -> (66.1667, -22.2222)
  line L136 (62.6667, -22.2222) -> (70.6667, -22.2222)
  line L137 (70.6667, -22.2222) -> (70.6667, -24.0741)
  line L138 (70.6667, -24.0741) -> (62.6667, -24.0741)
  line L139 (62.6667, -24.0741) -> (62.6667, -22.2222)
  line L140 (62.6667, -44.4444) -> (70.6667, -44.4444)
  line L141 (70.6667, -44.4444) -> (70.6667, -42.5926)
  line L142 (70.6667, -42.5926) -> (62.6667, -42.5926)
  line L143 (62.6667, -42.5926) -> (62.6667, -44.4444)
  dimension "d299" = 1
  dimension "d301" = 8
  dimension "d302" = 1.8519
  dimension "d303" = 1.8519
  dimension "d304" = 8
  dimension "d305" = 3.5
  dimension "d306" = 22.2222
  constraint horizontal L132
  constraint vertical L133
  constraint horizontal L134
  constraint vertical L135
  constraint coincident L57 L132.start
  constraint horizontal L136
  constraint vertical L137
  constraint horizontal L138
  constraint vertical L139
  constraint coincident L57.end L58.start
  constraint horizontal L140
  constraint vertical L141
  constraint horizontal L142
  constraint vertical L143
  constraint coincident L100.end L101.start
  measures "d299" distance of L133.end L134.end
  measures "d301" distance of L141.end L142.end
  measures "d302" distance of L100.end L142.end
  measures "d303" distance of L57.end L138.end
  measures "d304" distance of L137.end L138.end
  measures "d305" distance of L101.end L133
  measures "d306" distance of L132.end L133.end
extrude "Extrude35" cut sketch "Sketch65" against normal blind 4 contours L57 L135 L136 L138 L139 | L57 L132 L133 L135 L136 L138 | L57 L133 L136 L137 L138 | L133 L135 L138 L142 | L101 L133 L134 L135 L140 L142 | L101 L135 L140 L142 L143 | L101 L133 L140 L141 L142 bodies 13